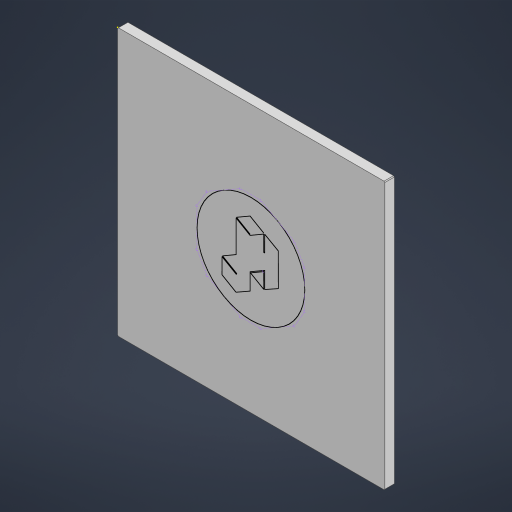
# Autodesk Inventor part: ScanCover
Saved by Autodesk Inventor 2023 (Build 270158000, 158)
## iProperties
Created: 2023-12-04
Part Number: ScanCover
Material: Generic
Document SubType Name: Modeling
Designer: FizzyApple12
Density: 1 g/cm^3
Appearance: Default
Author: FizzyApple12
Autodesk Inventor part; units mm, degrees
ref_plane "YZ Plane" through (0, 0, 0) normal (1, 0, 0) x (0, 1, 0)
ref_plane "XZ Plane" through (0, 0, 0) normal (0, 1, 0) x (-1, 0, 0)
ref_plane "XY Plane" through (0, 0, 0) normal (0, 0, 1) x (1, 0, 0)
sketch "Sketch1" plane through (0, 0, 0) normal (0, 0, 1) x (1, 0, 0)
  line L0 (0, 0) -> (84, 0)
  line L1 (84, 0) -> (84, -84)
  line L2 (84, -84) -> (0, -84)
  line L3 (0, -84) -> (0, 0)
  dimension "d0" = 84
  dimension "d1" = 84
  constraints: 8 end point, 2 parallel, 1 horizontal, 1 perpendicular
  measures "d0" distance of L1.end L2.end
  measures "d1" distance of L0.end L1.end
extrude "Extrusion1" add sketch "Sketch1" along normal blind 3
sketch "Sketch4" plane through (0, 0, 3) normal (0, 0, 1) x (1, 0, 0)
  line L0 (37.1993, -33.2294) -> (41.6014, -35.7961)
  line L1 (41.6014, -35.7961) -> (45.8654, -33.3061)
  line L2 (45.8654, -33.3061) -> (45.8781, -38.2734)
  line L3 (45.8781, -38.2734) -> (46.1686, -38.2768)
  line L4 (46.1686, -38.2768) -> (46.184, -33.1688)
  line L5 (46.184, -33.1688) -> (50.4528, -35.5818)
  line L6 (50.4528, -35.5818) -> (50.4793, -45.8437)
  line L7 (50.4793, -45.8437) -> (46.1838, -48.2415)
  line L8 (46.1838, -48.2415) -> (46.1838, -43.0247)
  line L9 (46.1838, -43.0247) -> (41.6014, -45.6918)
  line L10 (41.6014, -45.6918) -> (41.6014, -50.9599)
  line L11 (41.6014, -50.9599) -> (37.1784, -53.4769)
  line L12 (37.1784, -53.4769) -> (32.763, -50.9128)
  line L13 (32.763, -50.9128) -> (32.7791, -45.9754)
  line L14 (32.7791, -45.9754) -> (37.2675, -48.5495)
  line L15 (37.2675, -48.5495) -> (37.4003, -48.2932)
  line L16 (37.4003, -48.2932) -> (32.9437, -45.7029)
  line L17 (32.9437, -45.7029) -> (37.2048, -43.2163)
  line L18 (37.2048, -43.2163) -> (37.1993, -33.2294)
  spline S0 degree 3 poles (45.8868, -43.4973) (45.8887, -43.4963) (45.8911, -43.4963) (45.8929, -43.4973) knots 0 0 0 0 1 1 1 1
  line L19 (45.8868, -43.4973) -> (45.8887, -43.4963) construction
  line L20 (45.8887, -43.4963) -> (45.8911, -43.4963) construction
  line L21 (45.8911, -43.4963) -> (45.8929, -43.4973) construction
  spline S1 degree 3 poles (45.8929, -43.4973) (45.8948, -43.4984) (45.8961, -43.5005) (45.8961, -43.5026) knots 0 0 0 0 1 1 1 1
  line L22 (45.8929, -43.4973) -> (45.8948, -43.4984) construction
  line L23 (45.8948, -43.4984) -> (45.8961, -43.5005) construction
  line L24 (45.8961, -43.5005) -> (45.8961, -43.5026) construction
  line L25 (41.7369, -45.9267) -> (45.8961, -48.3358)
  line L26 (45.8961, -48.3358) -> (41.7369, -45.9267)
  line L27 (45.8961, -43.5026) -> (45.8961, -48.3358)
  line L28 (45.8961, -48.3358) -> (45.8837, -43.5132)
  line L29 (45.8837, -43.5132) -> (41.7369, -45.9267)
  line L30 (41.7369, -45.9267) -> (45.8929, -43.4973)
  line L31 (45.8929, -43.4973) -> (45.8961, -48.3358)
  line L32 (45.8961, -48.3358) -> (41.7369, -45.9267)
  spline S2 degree 3 poles (33.4713, -27.5312) (38.6612, -24.5702) (45.0282, -24.566) (50.2413, -27.52) knots 0 0 0 0 1 1 1 1
  line L33 (33.4713, -27.5312) -> (38.6612, -24.5702) construction
  line L34 (38.6612, -24.5702) -> (45.0282, -24.566) construction
  line L35 (45.0282, -24.566) -> (50.2413, -27.52) construction
  line L36 (41.6014, -35.4897) -> (37.3337, -33.0013)
  line L37 (37.3337, -33.0013) -> (41.5995, -30.5274)
  line L38 (41.5995, -30.5274) -> (45.8654, -32.9997)
  spline S3 degree 3 poles (50.4139, -27.6184) (55.5902, -30.5671) (58.7866, -36.0662) (58.7866, -42.0236) knots 0 0 0 0 1 1 1 1
  line L39 (50.4139, -27.6184) -> (55.5902, -30.5671) construction
  line L40 (55.5902, -30.5671) -> (58.7866, -36.0662) construction
  line L41 (58.7866, -36.0662) -> (58.7866, -42.0236) construction
  spline S4 degree 3 poles (58.7866, -42.0236) (58.7866, -47.981) (55.5902, -53.4801) (50.4139, -56.4288) knots 0 0 0 0 1 1 1 1
  line L42 (58.7866, -42.0236) -> (58.7866, -47.981) construction
  line L43 (58.7866, -47.981) -> (55.5902, -53.4801) construction
  line L44 (55.5902, -53.4801) -> (50.4139, -56.4288) construction
  line L45 (50.2413, -27.52) -> (50.4139, -27.6184)
  spline S5 degree 3 poles (50.2557, -56.5189) (45.0321, -59.4881) (38.6652, -59.4924) (33.4713, -56.5383) knots 0 0 0 0 1 1 1 1
  line L46 (50.2557, -56.5189) -> (45.0321, -59.4881) construction
  line L47 (45.0321, -59.4881) -> (38.6652, -59.4924) construction
  line L48 (38.6652, -59.4924) -> (33.4713, -56.5383) construction
  line L49 (50.4139, -56.4288) -> (50.2557, -56.5189)
  spline S6 degree 3 poles (33.2987, -56.44) (28.1224, -53.4912) (24.926, -47.9921) (24.926, -42.0348) knots 0 0 0 0 1 1 1 1
  line L50 (33.2987, -56.44) -> (28.1224, -53.4912) construction
  line L51 (28.1224, -53.4912) -> (24.926, -47.9921) construction
  line L52 (24.926, -47.9921) -> (24.926, -42.0348) construction
  spline S7 degree 3 poles (24.926, -42.0348) (24.926, -36.0774) (28.1224, -30.5783) (33.2987, -27.6295) knots 0 0 0 0 1 1 1 1
  line L53 (24.926, -42.0348) -> (24.926, -36.0774) construction
  line L54 (24.926, -36.0774) -> (28.1224, -30.5783) construction
  line L55 (28.1224, -30.5783) -> (33.2987, -27.6295) construction
  line L56 (33.4713, -56.5383) -> (33.2987, -56.44)
  line L57 (33.2987, -27.6295) -> (33.4713, -27.5312)
  point P0 (0, 0)
  constraints: 68 end point, 5 parallel, 1 vertical, 28 other
chamfer "Chamfer1" distance 0.25 angle 45 4 edges at (0, 0, 1.5) (84, 0, 1.5) (84, -84, 1.5) (0, -84, 1.5)
body "Solid1"
